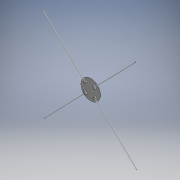
# Autodesk Inventor part: Spinning Platform
Saved by Autodesk Inventor 2016 (Build 200138000, 138)
## iProperties
Created: 2015-12-21
Part Number: Spinning Platform
Material: Generic
Document SubType Name: Modeling
Designer: jonathan
Density: 1 g/cm^3
Appearance: Default
Author: jonathan
Autodesk Inventor part; units mm, degrees
ref_plane "YZ Plane" through (0, 0, 0) normal (1, 0, 0) x (0, 1, 0)
ref_plane "XZ Plane" through (0, 0, 0) normal (0, 1, 0) x (-1, 0, 0)
ref_plane "XY Plane" through (0, 0, 0) normal (0, 0, 1) x (1, 0, 0)
sketch "Sketch1" plane through (0, 0, 0) normal (0, 1, 0) x (-1, 0, 0)
  circle A0 centre (0, 0) radius 70
  dimension "d0" = 140
  constraints: 1 centre point, 1 coincident
  measures "d0" diameter of A0
extrude "Extrusion1" add sketch "Sketch1" along normal blind 1
sketch "Sketch2" plane through (0, 0, 0) normal (0, -1, 0) x (1, 0, 0)
  line L0 (0, 0) -> (36.3053, 37.4305)
  line L1 (36.3053, 37.4305) -> (28.3938, 45.1042)
  line L2 (28.3938, 45.1042) -> (20.7201, 37.1927)
  line L3 (20.7201, 37.1927) -> (28.6316, 29.519)
  line L4 (36.5432, 21.8453) -> (44.2169, 29.7568)
  line L5 (44.2169, 29.7568) -> (36.3053, 37.4305)
  line L6 (28.6316, 29.519) -> (36.5432, 21.8453)
  constraints: 14 end point, 5 perpendicular, 3 point on line, 2 equal length
extrude "Extrusion2" add sketch "Sketch2" along normal blind 10
sketch "Sketch3" plane through (28.3938, -10, 45.1042) normal (0.6962355, 0, 0.7178134) x (0.7178134, 0, -0.6962355)
  circle A0 centre (11.0217, 5.114) radius 2.5
  point P0 (11.0217, 10)
  dimension "d5" = 5
  constraints: 1 centre point
  measures "d5" diameter of A0
extrude "Extrusion3" add sketch "Sketch3" along normal blind 418.75
pattern_circular "Circular Pattern1" count 4 over 360 about axis through (0, 0, 0) along (0, 1, 0) of "Extrusion2", "Extrusion3"
body "Solid1"
